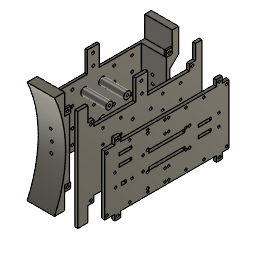
soccerbot (Autodesk Fusion 360 design; units mm, degrees)
part number: 2026-01-25-12-54-34-821
Autodesk Fusion 360 part; units mm, degrees
sketch "Sketch1" plane through (0, 0, 0) normal (1, 0, 0) x (0, 1, 0)
sketch "Base FL1" plane through (0, 0, 0) normal (1, 0, 0) x (0, 1, 0)
  line L0 (176.22, 50.0312) -> (1.6941, 50.0085) construction
  line L1 (90, 0) -> (90, 99.9394) construction
  line L2 (40, 22) -> (140, 22) construction
  line L3 (155, 34) -> (125, 34)
  line L4 (125, 34) -> (125, 10)
  line L5 (125, 10) -> (155, 10)
  line L6 (155, 10) -> (155, 34)
  line L7 (154.9958, 66.0568) -> (124.9958, 66.049)
  line L8 (124.9958, 66.049) -> (124.9896, 90.049)
  line L9 (124.9896, 90.049) -> (154.9896, 90.0568)
  line L10 (154.9896, 90.0568) -> (154.9958, 66.0568)
  line L11 (55, 34) -> (55, 10)
  line L12 (25, 34) -> (55, 34)
  line L13 (25, 10) -> (25, 34)
  line L14 (55, 10) -> (25, 10)
  line L15 (124.9896, 90.049) -> (154.9896, 90.0568)
  line L16 (124.9958, 66.049) -> (124.9896, 90.049)
  line L17 (154.9896, 90.0568) -> (154.9958, 66.0568)
  line L18 (154.9958, 66.0568) -> (124.9958, 66.049)
  line L19 (54.9896, 90.0308) -> (24.9896, 90.023)
  line L20 (54.9958, 66.0308) -> (54.9896, 90.0308)
  line L21 (24.9958, 66.023) -> (54.9958, 66.0308)
  line L22 (24.9896, 90.023) -> (24.9958, 66.023)
  line L23 (140, 10) -> (140, -25) construction
  line L24 (175, -25) -> (105, -25) construction
  line L25 (100, 0) -> (86, 0)
  line L26 (100, -35) -> (100, 0)
  line L27 (80, -35) -> (80, 0)
  line L28 (180, -35) -> (191, -35)
  line L29 (191, 135) -> (180, 135)
  line L30 (0, -36.9171) -> (-17, -36.8837)
  line L31 (5, -25) -> (75, -25) construction
  line L32 (191, 135) -> (191, 95)
  circle A0 centre (105, 22) radius 6
  circle A1 centre (75, 22) radius 6
  circle A2 centre (74.9927, 78.036) radius 6
  circle A3 centre (105.0073, 78.036) radius 6
  line L33 (180, 0) -> (0, 0)
  line L34 (176.2425, 80.55) -> (176.1975, 19.5123)
  line L35 (180, 0) -> (180, -35)
  line L36 (0, 0) -> (0, -36.9171)
  line L37 (180, 100) -> (0, 100)
  line L38 (180, 135) -> (180, 100)
  line L39 (176.1975, 19.5123) -> (191, 5)
  line L40 (191, 5) -> (191, -35)
  line L41 (191, 95) -> (176.2425, 80.55)
  line L42 (4.9805, 125.0178) -> (74.9805, 125.036) construction
  line L43 (174.9805, 125.062) -> (104.9805, 125.0438) construction
  line L44 (0, 100) -> (0, 135)
  line L45 (0, 135) -> (-17, 135)
  arc A4 (-17, -36.8837) -> (-17, 135) centre (-205.1779, 49.0581) ccw
  line L46 (8.1772, 100) -> (8.1772, 0)
  line L47 (170.3633, 100) -> (170.3633, 0)
  line L48 (100, 100) -> (100, 135)
  line L49 (80, 100) -> (80, 135)
  line L50 (100, 135) -> (80, 135)
  line L51 (80, -35) -> (100, -35)
  point P0 (90, 22)
  point P1 (40, 22)
  point P2 (39.9927, 78.0269)
  point P3 (39.9927, 78.0269)
  point P4 (176.1975, 19.5123)
  point P5 (191, 5)
  dimension "d2" = 180
  dimension "d31" = 30
  dimension "d32" = 30
  dimension "d33" = 24
  dimension "d36" = 35
  dimension "d46" = 17
  dimension "d47" = 11
  dimension "d51" = 12
  dimension "d53" = 11
  dimension "d59" = 35
  dimension "d63" = 35
  dimension "d64" = 17
  dimension "d65" = 35
  dimension "d66" = 35
  constraint midpoint L2 P0
  constraint coincident L1 P0
  constraint perpendicular L1 L2
  constraint horizontal L3
  constraint vertical L4
  constraint horizontal L5
  constraint vertical L6
  constraint symmetric L0 L3.start L7.start
  constraint symmetric L0 L3.end L7.end
  constraint symmetric L0 L4.end L8.end
  constraint symmetric L0 L5.end L9.end
  constraint symmetric L1 L2.end P1
  constraint symmetric L1 L3.start L12.start
  constraint symmetric L1 L3.end L11.start
  constraint symmetric L1 L4.end L11.end
  constraint symmetric L1 L5.end L13.start
  constraint symmetric L0 P1 P3
  constraint symmetric L0 L11.end L19.start
  constraint symmetric L0 L11.start L20.start
  constraint symmetric L0 L13.start L19.end
  constraint symmetric L0 L12.start L21.start
  constraint midpoint L5 L23.start
  constraint perpendicular L5 L23
  constraint midpoint L23.end L24
  constraint perpendicular L23 L24
  constraint horizontal L25
  constraint vertical L26
  constraint symmetric L1 L25.start L27.end
  constraint symmetric L1 L26.start L27.start
  constraint horizontal L28
  constraint horizontal L29
  constraint symmetric L1 L24.start L31.start
  constraint symmetric L1 L24.end L31.end
  constraint coincident L2 A0.centre
  constraint symmetric L1 A0 A1
  constraint symmetric L0 A1 A2
  constraint symmetric L1 A2 A3
  constraint coincident L33.end L36.start
  constraint vertical L36
  constraint horizontal L37
  constraint coincident P4 L34.end
  constraint coincident P5 L39.end
  constraint vertical L32
  constraint symmetric L0 L31.start L42.start
  constraint symmetric L0 L31.end L42.end
  constraint symmetric L0 L24.start L43.start
  constraint symmetric L0 L24.end L43.end
  constraint perpendicular L37 L44
  constraint perpendicular L44 L45
  constraint coincident L0.end A4
  constraint midpoint L0.start L34
  constraint coincident L37 L46.start
  constraint coincident L33 L46.end
  constraint perpendicular L33 L46
  constraint coincident L37 L47.start
  constraint coincident L33 L47.end
  constraint perpendicular L33 L47
  constraint coincident L37 L48.start
  constraint perpendicular L37 L48
  constraint coincident L37 L49.start
  constraint perpendicular L37 L49
  constraint perpendicular L26 L51
  measures "d2" distance of L33.end L33.start
  measures "d31" distance of L4.end L5.end
  measures "d32" distance of L3.start L3.end
  measures "d33" distance of L3.start L5.end
  measures "d36" distance of L25.start L26.start
  measures "d46" distance of L30.end L30.start
  measures "d47" distance of L28.start L28.end
  measures "d51" diameter of A0
  measures "d53" distance of L29.start L29.end
  measures "d59" distance of L33.start L28.start
  measures "d63" distance of L37.end L44.end
  measures "d64" distance of L44.end L45.end
  measures "d65" distance of L48.start L48.end
  measures "d66" distance of L49.start L49.end
extrude "Extrude4" add sketch "Base FL1" along normal blind 46 contours L28 L29 L32 L33 L34 L35 L37 L38 L39 L40 L41 L47 | L30 L33 L36 L37 L44 L45 A4 L46 | A0 | A1 | A2 | A3 makes body 1 at (30.6667, 69.0225, 77.4386) makes body 2 at (30.6667, 0.7595, 68.7236) makes body 3 at (30.6667, 80.9925, 21.7009) makes body 4 at (30.6667, 99.0371, 77.4386) makes body 5 at (30.6667, 170.3633, 66.6667) makes body 6 at (30.6667, 110.9925, 21.7009)
extrude "Extrude5" add sketch "Base FL1" along normal blind 4 contours L3 L4 L5 L6 | L7 L8 L9 L10 L15 L16 L17 L18 | L11 L12 L13 L14 | L19 L20 L21 L22 | L25 L26 L27 L33 L51 | L25 L33 L37 L46 L47 | L37 L48 L49 L50 bodies 1 2 3 4 5 6
hole "Hole3" at (0, 25, 10) at (0, 25, 34) at (0, 55, 34) at (0, 55, 10) at (0, 125, 34) at (0, 155, 34) at (0, 155, 10) at (0, 125, 10) at (0, 124.9896, 90.049) at (0, 154.9896, 90.0568) at (0, 154.9958, 66.0568) at (0, 124.9958, 66.049) at (0, 54.9958, 66.0308) at (0, 54.9896, 90.0308) at (0, 24.9896, 90.023) at (0, 24.9958, 66.023) direction (1, 0, 0) diameter 4.5 depth 4 tip angle 180 bodies 1
hole "Hole4" at (0, 74.9927, 78.036) at (0, 105.0073, 78.036) at (0, 105, 22) at (0, 75, 22) direction (1, 0, 0) diameter 3.783 depth 20 tip angle 180 bodies 1
thread "Thread1" "ISO Metric profile 4.5 M4.5x0.75 M4.5x0.75 6H" major diameter 4.6131 minor diameter 3.7831 pitch 0.75 angle 60 resizes the face on face at (6.6667, 106.5431, 76.9319) on face at (6.6667, 105.0943, 23.8891) on face at (6.6667, 76.5285, 76.9319) on face at (6.6667, 75.0943, 23.8891) on bodies 1
hole "Hole5" at (0, 74.9927, 78.036) at (0, 105.0073, 78.036) at (0, 105, 22) at (0, 75, 22) direction (1, 0, 0) diameter 3.783 depth 46 tip angle 180 bodies 1
thread "Thread2" "ISO Metric profile 4.5 M4.5x0.75 M4.5x0.75 6H" major diameter 4.6131 minor diameter 3.7831 pitch 0.75 angle 60 resizes the face on face at (28.6667, 75.1883, 23.8821) on face at (28.6667, 76.5816, 77.0098) on face at (28.6667, 105.1883, 23.8821) on face at (28.6667, 106.5962, 77.0098) on bodies 1
hole "Hole6" at (4, 89.3779, 126.1811) direction (-1, 0, 0) diameter 4.5 depth 4 tip angle 180 bodies 1
hole "Hole7" at (4, 90.0772, 107.2797) direction (-1, 0, 0) diameter 4.5 depth 4 tip angle 180 bodies 1
hole "Hole8" at (22.4648, 176.2297, 63.2035) direction (0, -1, 0.000737) diameter 4.5 depth 5.877 tip angle 180 bodies 1
hole "Hole9" at (23, 176.22, 50.0312) direction (0, -1, 0.000737) diameter 4.5 depth 5.877 tip angle 180 bodies 1
hole "Hole10" at (23.0599, 176.2099, 36.3846) direction (0, -1, 0.000737) diameter 4.5 depth 5.877 tip angle 180 bodies 1
hole "Hole11" at (15.3916, 74.9927, 76.1445) direction (0, 0, -1) diameter 4.5 depth 5.877 tip angle 180 bodies 1
hole "Hole12" at (11.1565, 105.0073, 76.1445) direction (0, 0, -1) diameter 4.5 depth 5.877 tip angle 180 bodies 1
hole "Hole13" at (23.1083, 8.1772, 51.0089) direction (0, -1, 0) diameter 4.5 depth 19 tip angle 180 bodies 1
hole "Hole14" at (22.5371, 8.1772, 33.9979) direction (0, -1, 0) diameter 4.5 depth 19 tip angle 180 bodies 1
hole "Hole15" at (22.1531, 8.1772, 69.5516) direction (0, -1, 0) diameter 4.5 depth 19 tip angle 180 bodies 1
hole "Hole16" at (4, 90.9402, 50.4012) direction (-1, 0, 0) diameter 4.5 depth 19 tip angle 180 bodies 1
hole "Hole17" at (4, 90.6117, -26.9418) direction (-1, 0, 0) diameter 4.5 depth 19 tip angle 180 bodies 1
hole "Hole18" at (4, 90.6117, -8.1238) direction (-1, 0, 0) diameter 4.5 depth 19 tip angle 180 bodies 1
sketch "Overhang 1" plane through (0, 0, 0) normal (0, 1, 0) x (-1, 0, 0)
  line L0 (0, 100) -> (0, 135)
  line L1 (0, 135) -> (-46, 135)
  line L2 (-46, 135) -> (-46, 100)
  line L3 (-46, 100) -> (0, 100)
  line L4 (-46, 110.0202) -> (-26, 110.0202)
  line L5 (-26, 100.0202) -> (-46, 100.0202)
  line L6 (-46, 100.0202) -> (-46, 110.0202)
  line L7 (-46, 110.0202) -> (-46, 109.0202)
  line L8 (-46, 100.0202) -> (-46, 101.0202)
  line L9 (-46, 100.0202) -> (-43, 100.0202)
  line L10 (-46, 100.0202) -> (-43, 100.0202)
  line L11 (-43, 100.0202) -> (-43, 110.0202)
  dimension "d124" = 20
  dimension "d125" = 10
  dimension "d126" = 1
  dimension "d127" = 1
  constraint horizontal L4
  constraint horizontal L5
  constraint vertical L6
  constraint coincident L2 L4.start
  constraint coincident L6 L7.end
  constraint coincident L6 L8.end
  constraint coincident L5 L9.end
  constraint coincident L4 L11.end
  constraint perpendicular L4 L11
  measures "d124" distance of L5.start L5.end
  measures "d125" distance of L4.start L5.end
  measures "d126" distance of L4.start L7.end
  measures "d127" distance of L5.end L8.end
extrude "Extrude6" add sketch "Overhang 1" along normal blind 10 separate body contours L2 L4 L5 L6 L7 L8 L9 L10 L11 makes body 7
sketch "Overhang 2" plane through (0, 0, 0) normal (0, 1, 0) x (-1, 0, 0)
  line L0 (0, -36.9171) -> (0, 0)
  line L1 (0, 0) -> (-46, 0)
  line L2 (-46, 0) -> (-46, -36.9171)
  line L3 (-46, -36.9171) -> (0, -36.9171)
  line L4 (-46, 0) -> (-43, 0)
  line L5 (-43, 0) -> (-43, -10)
  line L6 (-43, -10) -> (-46, -10)
  line L7 (-46, -10) -> (-46, 0)
  dimension "d130" = 10
  dimension "d131" = 3
  constraint horizontal L4
  constraint vertical L5
  constraint horizontal L6
  constraint vertical L7
  constraint coincident L1.end L2.start
  measures "d130" distance of L4.end L5.end
  measures "d131" distance of L5.end L6.end
extrude "Extrude7" add sketch "Overhang 2" along normal blind 10 separate body contours L1 L2 L4 L5 L6 L7 makes body 8
sketch "Overhang 3 - 4" plane through (0, 180, 0) normal (0, -1, 0) x (1, 0, 0)
  line L0 (0, 135) -> (0, 100)
  line L1 (0, 100) -> (46, 100)
  line L2 (46, 100) -> (46, 135)
  line L3 (46, 135) -> (0, 135)
  line L4 (46, 110.1305) -> (46, 100.1305)
  line L5 (46, -10) -> (46, 0)
  line L6 (46, 0) -> (43, 0)
  line L7 (43, 0) -> (43, -10)
  line L8 (43, -10) -> (46, -10)
  line L9 (46, -10) -> (46, 0)
  line L10 (46, 100) -> (43, 100)
  line L11 (43, 100) -> (43, 110)
  line L12 (43, 110) -> (46, 110)
  line L13 (46, 110) -> (46, 100)
  point P0 (46, 0)
  dimension "d144" = 10
  dimension "d145" = 3
  constraint vertical L4
  constraint coincident L2 L4.end
  constraint vertical L5
  constraint horizontal L6
  constraint vertical L7
  constraint horizontal L8
  constraint vertical L9
  constraint coincident P0 L5.end
  constraint horizontal L10
  constraint vertical L11
  constraint horizontal L12
  constraint vertical L13
  constraint coincident L1.end L2.start
  measures "d144" distance of L1.end L12.end
  measures "d145" distance of L1.end L10.end
extrude "Extrude8" add sketch "Overhang 3 - 4" along normal blind 10 separate body contours L5 L6 L7 L8 L9 makes body 9
extrude "Extrude10" add sketch "Overhang 3 - 4" along normal blind 10 separate body contours L1 L2 L4 L10 L11 L12 L13 makes body 10
hole "Hole19" at (46, 174.9154, 104.8549) direction (-1, 0, 0) diameter 4.5 end through all bodies 10
hole "Hole20" at (46, 175.0929, -5) direction (-1, 0, 0) diameter 4.5 depth 3 tip angle 180 bodies 9
hole "Hole21" at (46, 5, -4.7674) direction (-1, 0, 0) diameter 4.5 depth 3 tip angle 180 bodies 8
hole "Hole22" at (46, 5, 105.2643) direction (-1, 0, 0) diameter 4.5 depth 3 tip angle 180 bodies 7
sketch "Base FL2" plane through (0, 0, 0) normal (1, 0, 0) x (0, 1, 0)
  line L0 (55, 34) -> (55, 10)
  line L1 (191, 50) -> (-17, 50) construction
  line L2 (55, 10) -> (25, 10)
  line L3 (25, 10) -> (25, 34)
  line L4 (124.9896, 90.049) -> (154.9896, 90.0568)
  line L5 (80, 100) -> (80, 135)
  line L6 (100, -35) -> (100, 0)
  line L7 (154.9896, 90.0568) -> (154.9958, 66.0568)
  line L8 (25, 34) -> (55, 34)
  line L9 (54.9896, 90.0308) -> (24.9896, 90.023)
  line L10 (125, 10) -> (155, 10)
  line L11 (154.9958, 66.0568) -> (124.9958, 66.049)
  line L12 (154.9958, 66.0568) -> (124.9958, 66.049)
  line L13 (54.9958, 66.0308) -> (54.9896, 90.0308)
  line L14 (154.9896, 90.0568) -> (154.9958, 66.0568)
  line L15 (100, 135) -> (80, 135)
  line L16 (24.9896, 90.023) -> (24.9958, 66.023)
  line L17 (155, 10) -> (155, 34)
  line L18 (180, 0) -> (180, -35)
  line L19 (100, 100) -> (100, 135)
  line L20 (125, 34) -> (125, 10)
  line L21 (180, -35) -> (191, -35)
  line L22 (124.9896, 90.049) -> (154.9896, 90.0568)
  line L23 (124.9958, 66.049) -> (124.9896, 90.049)
  line L24 (180, 135) -> (180, 100)
  line L25 (124.9958, 66.049) -> (124.9896, 90.049)
  line L26 (80, -35) -> (100, -35)
  line L27 (80, -35) -> (80, 0)
  line L28 (24.9958, 66.023) -> (54.9958, 66.0308)
  line L29 (0, 135) -> (0, 100)
  line L30 (170, 0) -> (170, -10)
  line L31 (170, -10) -> (180, -10)
  line L32 (191, -35) -> (191, 135)
  line L33 (191, 135) -> (180, 135)
  line L34 (180, 135) -> (180, 110)
  line L35 (170, 100) -> (170, 110)
  line L36 (170, 110) -> (180, 110)
  line L37 (0, 110) -> (10, 110)
  line L38 (10, 110) -> (10, 100)
  line L39 (125, 34) -> (125, 10)
  line L40 (155, 10) -> (155, 34)
  line L41 (0, 135) -> (-17, 135)
  line L42 (125, 34) -> (155, 34)
  line L43 (180, 100) -> (100, 100)
  line L44 (0, 100) -> (80, 100)
  line L45 (0, 0) -> (80, 0)
  line L46 (0, 0.2133) -> (0, -34.7867)
  line L47 (0, -34.7867) -> (-17, -34.7867)
  line L48 (-17, 135) -> (-17, -34.7867)
  line L49 (180, 0) -> (100, 0)
  line L50 (0, -10) -> (10, -10)
  line L51 (10, -10) -> (10, 0)
  line L52 (24.9927, 59.9133) -> (55, 59.9133)
  line L53 (55, 59.9133) -> (55, 40)
  line L54 (55, 40) -> (24.9927, 40)
  line L55 (24.9927, 40) -> (24.9927, 59.9133)
  line L56 (90, 135) -> (90, -35) construction
  line L57 (155.0073, 59.9133) -> (125, 59.9133)
  line L58 (125, 59.9133) -> (125, 40)
  line L59 (125, 40) -> (155.0073, 40)
  line L60 (155.0073, 40) -> (155.0073, 59.9133)
  circle A0 centre (105.0073, 78.036) radius 6
  circle A1 centre (105.0073, 21.964) radius 6
  circle A2 centre (74.9927, 21.964) radius 6
  line L61 (180, 0) -> (180, -35)
  line L62 (155, 10) -> (155, 34)
  line L63 (155.0073, 40) -> (155.0073, 59.9133)
  line L64 (-17, 135) -> (-17, -34.7867)
  line L65 (80, -35) -> (100, -35)
  line L66 (54.9896, 90.0308) -> (24.9896, 90.023)
  line L67 (55, 10) -> (25, 10)
  line L68 (155, 10) -> (155, 34)
  line L69 (125, 40) -> (155.0073, 40)
  line L70 (170, 0) -> (170, -10)
  line L71 (24.9927, 59.9133) -> (55, 59.9133)
  line L72 (155.0073, 59.9133) -> (125, 59.9133)
  line L73 (154.9958, 66.0568) -> (124.9958, 66.049)
  line L74 (124.9896, 90.049) -> (154.9896, 90.0568)
  line L75 (124.9896, 90.049) -> (154.9896, 90.0568)
  line L76 (124.9958, 66.049) -> (124.9896, 90.049)
  line L77 (0, 135) -> (0, 100)
  line L78 (25, 34) -> (55, 34)
  line L79 (0, 110) -> (10, 110)
  line L80 (154.9896, 90.0568) -> (154.9958, 66.0568)
  line L81 (180, 135) -> (180, 100)
  line L82 (125, 34) -> (125, 10)
  line L83 (170, -10) -> (180, -10)
  line L84 (124.9958, 66.049) -> (124.9896, 90.049)
  line L85 (0, 0) -> (80, 0)
  line L86 (191, 135) -> (180, 135)
  line L87 (10, 110) -> (10, 100)
  line L88 (80, -35) -> (80, 0)
  line L89 (0, 100) -> (80, 100)
  line L90 (0, 135) -> (-17, 135)
  line L91 (100, -35) -> (100, 0)
  line L92 (55, 40) -> (24.9927, 40)
  line L93 (125, 10) -> (155, 10)
  line L94 (170, 100) -> (170, 110)
  line L95 (154.9958, 66.0568) -> (124.9958, 66.049)
  line L96 (125, 34) -> (155, 34)
  line L97 (125, 34) -> (125, 10)
  line L98 (170, 110) -> (180, 110)
  line L99 (24.9958, 66.023) -> (54.9958, 66.0308)
  line L100 (55, 34) -> (55, 10)
  line L101 (180, -35) -> (191, -35)
  line L102 (180, 135) -> (180, 110)
  line L103 (80, 100) -> (80, 135)
  line L104 (100, 100) -> (100, 135)
  circle A3 centre (74.9927, 78.036) radius 6
  line L105 (100, 135) -> (80, 135)
  line L106 (24.9896, 90.023) -> (24.9958, 66.023)
  line L107 (54.9958, 66.0308) -> (54.9896, 90.0308)
  line L108 (191, 50) -> (-17, 50) construction
  line L109 (25, 10) -> (25, 34)
  line L110 (10, -10) -> (10, 0)
  line L111 (0, 0.2133) -> (0, -34.7867)
  line L112 (180, 0) -> (100, 0)
  line L113 (0, -10) -> (10, -10)
  line L114 (0, -34.7867) -> (-17, -34.7867)
  line L115 (125, 59.9133) -> (125, 40)
  line L116 (90, 135) -> (90, -35) construction
  line L117 (191, -35) -> (191, 135)
  line L118 (180, 100) -> (100, 100)
  line L119 (24.9927, 40) -> (24.9927, 59.9133)
  line L120 (55, 59.9133) -> (55, 40)
  circle A4 centre (25, 34) radius 2
  circle A5 centre (25, 10) radius 2
  circle A6 centre (55, 34) radius 2
  circle A7 centre (55, 10) radius 2
  circle A8 centre (24.9896, 90.023) radius 2
  circle A9 centre (54.9896, 90.0308) radius 2
  circle A10 centre (54.9958, 66.0308) radius 2
  circle A11 centre (24.9958, 66.023) radius 2
  circle A12 centre (74.9927, 21.964) radius 6
  circle A13 centre (105.0073, 21.964) radius 6
  circle A14 centre (105.0073, 78.036) radius 6
  circle A15 centre (74.9927, 78.036) radius 6
  circle A16 centre (124.9958, 66.049) radius 2
  circle A17 centre (154.9958, 66.0568) radius 2
  circle A18 centre (154.9896, 90.0568) radius 2
  circle A19 centre (124.9896, 90.049) radius 2
  circle A20 centre (155, 34) radius 2
  circle A21 centre (155, 10) radius 2
  circle A22 centre (125, 10) radius 2
  circle A23 centre (125, 34) radius 2
  dimension "d237" = 4
  dimension "d238" = 4
  dimension "d239" = 4
  dimension "d240" = 4
  dimension "d241" = 4
  dimension "d242" = 4
  dimension "d243" = 4
  dimension "d244" = 4
  dimension "d245" = 12
  dimension "d246" = 12
  dimension "d247" = 12
  dimension "d248" = 4
  dimension "d249" = 4
  dimension "d250" = 4
  dimension "d251" = 4
  dimension "d252" = 4
  dimension "d253" = 4
  dimension "d254" = 4
  dimension "d255" = 4
  constraint coincident L18 L31.end
  constraint coincident L24 L34.end
  constraint coincident L29 L37.start
  constraint perpendicular L29 L37
  constraint perpendicular L17 L42
  constraint midpoint L1.start L32
  constraint coincident L45.start L85.start
  constraint perpendicular L27 L45
  constraint perpendicular L45 L46
  constraint perpendicular L46 L47
  constraint perpendicular L6 L49
  constraint coincident L46 L50.start
  constraint perpendicular L46 L50
  constraint coincident L45 L51.end
  constraint perpendicular L45 L51
  constraint horizontal L52
  constraint vertical L53
  constraint horizontal L54
  constraint vertical L55
  constraint midpoint L15 L56.start
  constraint midpoint L26 L56.end
  constraint symmetric L52.start L56 L57.start
  constraint symmetric L52.end L56 L57.end
  constraint symmetric L53.end L56 L58.end
  constraint symmetric L54.end L56 L59.end
  constraint symmetric L1 A0 A1
  constraint symmetric L56 A1 A2
  constraint coincident L31.end L61
  constraint coincident L34.end L81
  constraint coincident L37.start L77
  constraint perpendicular L77 L79
  constraint perpendicular L68 L96
  constraint midpoint L1.start L117
  constraint perpendicular L85 L88
  constraint perpendicular L85 L111
  constraint perpendicular L111 L114
  constraint perpendicular L91 L112
  constraint coincident L50.start L111
  constraint perpendicular L111 L113
  constraint coincident L51.end L85
  constraint perpendicular L85 L110
  constraint horizontal L71
  constraint vertical L120
  constraint horizontal L92
  constraint vertical L119
  constraint midpoint L56.start L105
  constraint midpoint L56.end L65
  constraint symmetric L57.start L52.start L116
  constraint symmetric L57.end L52.end L116
  constraint symmetric L58.end L53.end L116
  constraint symmetric L54.end L59.end L116
  constraint coincident L3.end L8.start
  constraint coincident L2.end L3.start
  constraint coincident L0.start L8.end
  constraint coincident L0.end L2.start
  constraint coincident L9.end L16.start
  constraint coincident L9.start L13.end
  constraint coincident L13.start L28.end
  constraint coincident L16.end L28.start
  constraint concentric A2 A12
  constraint concentric A1 A13
  constraint concentric A0 A14
  constraint concentric A3 A15
  constraint coincident L11.end L12.end
  constraint coincident L7.end L11.start
  constraint coincident L4.end L7.start
  constraint coincident L4.start L22.start
  constraint coincident L17.end L40.end
  constraint coincident L10.end L17.start
  constraint coincident L10.start L20.end
  constraint coincident L20.start L39.start
  measures "d237" diameter of A7
  measures "d238" diameter of A6
  measures "d239" diameter of A4
  measures "d240" diameter of A5
  measures "d241" diameter of A11
  measures "d242" diameter of A8
  measures "d243" diameter of A9
  measures "d244" diameter of A10
  measures "d245" diameter of A14
  measures "d246" diameter of A13
  measures "d247" diameter of A12
  measures "d248" diameter of A22
  measures "d249" diameter of A21
  measures "d250" diameter of A20
  measures "d251" diameter of A23
  measures "d252" diameter of A16
  measures "d253" diameter of A17
  measures "d254" diameter of A18
  measures "d255" diameter of A19
sketch "Sketch8" plane through (55, 0, 0) normal (1, 0, 0) x (0, 1, 0)
extrude "Extrude12" add sketch "Base FL2" along normal blind 5 separate body contours L0 L2 L3 L8 L67 L78 L100 L109 A4 A5 A6 A7 | L4 L7 L11 L12 L14 L22 L23 L25 L73 L74 L75 L76 L80 L84 L95 A16 A17 A18 A19 | L5 L6 L15 L18 L19 L21 L24 L26 L27 L29 L32 L33 L34 L41 L43 L44 L45 L46 L47 L48 L49 L61 L64 L65 L77 L81 L85 L86 L88 L89 L90 L91 L101 L102 L103 L104 L105 L111 L112 L114 L117 L118 | L29 L37 L38 L44 L77 L79 L87 L89 | L24 L35 L36 L43 L81 L94 L98 L118 | L45 L46 L50 L51 L85 L110 L111 L113 | L18 L30 L31 L49 L61 L70 L83 L112 | L9 L13 L16 L28 L66 L99 L106 L107 A8 A9 A10 A11 | L10 L17 L20 L39 L40 L42 L62 L68 L82 L93 L96 L97 A20 A21 A22 A23 | A0 A14 | A1 A13 | A2 A12 | A3 A15 makes body 11
hole "Hole35" at (0, 74.9927, 78.036) direction (1, 0, 0) diameter 4.5 depth 5 tip angle 180 bodies 11
hole "Hole36" at (0, 105.0073, 78.036) direction (1, 0, 0) diameter 4.5 depth 5 tip angle 180 bodies 11
hole "Hole37" at (0, 105.0073, 21.964) direction (1, 0, 0) diameter 4.5 depth 5 tip angle 180 bodies 11
hole "Hole38" at (0, 74.9927, 21.964) direction (1, 0, 0) diameter 4.5 depth 5 tip angle 180 bodies 11
move_body "Move2" bodies 11 to x (1, 0, 0) y (0, 1, 0) z (0, 0, 1) at (50, 0, 0)
hole "Hole39" at (50, 174.9118, 104.9201) direction (1, 0, 0) diameter 4.5 depth 5 tip angle 180 bodies 11
hole "Hole40" at (50, 175.1424, -5.038) direction (1, 0, 0) diameter 4.5 depth 5 tip angle 180 bodies 11
hole "Hole41" at (50, 90.3269, -8.1207) direction (1, 0, 0) diameter 4.5 depth 5 tip angle 180 bodies 11
hole "Hole42" at (50, 90.6224, -26.9185) direction (1, 0, 0) diameter 4.5 depth 5 tip angle 180 bodies 11
hole "Hole43" at (50, 90.9577, 50.4083) direction (1, 0, 0) diameter 4.5 depth 5 tip angle 180 bodies 11
hole "Hole44" at (50, 89.3921, 126.1895) direction (1, 0, 0) diameter 4.5 depth 5 tip angle 180 bodies 11
hole "Hole45" at (50, 90.0893, 107.3095) direction (1, 0, 0) diameter 4.5 depth 5 tip angle 180 bodies 11
hole "Hole46" at (50, 5.0185, -4.7346) direction (1, 0, 0) diameter 4.5 depth 5 tip angle 180 bodies 11
hole "Hole47" at (50, 5.0143, 105.2605) direction (1, 0, 0) diameter 4.5 depth 5 tip angle 180 bodies 11
sketch "Sketch9" plane through (55, 0, 0) normal (1, 0, 0) x (0, 1, 0)
  line L0 (-17.0199, 0) -> (190.9801, 0)
  line L1 (190.9801, 0) -> (190.9801, 100)
  line L2 (190.9801, 100) -> (-17.0199, 100)
  line L3 (-17.0199, 100) -> (-17.0199, 0)
  line L4 (0, 100) -> (10, 100)
  line L5 (10, 100) -> (10, 110)
  line L6 (10, 110) -> (0, 110)
  line L7 (0, 110) -> (0, 100)
  line L8 (0, 0) -> (10, 0)
  line L9 (10, 0) -> (10, -10)
  line L10 (10, -10) -> (0, -10)
  line L11 (0, -10) -> (0, 0)
  line L12 (180, 0) -> (170, 0)
  line L13 (170, 0) -> (170, -10)
  line L14 (170, -10) -> (180, -10)
  line L15 (180, -10) -> (180, 0)
  line L16 (180, 100) -> (170, 100)
  line L17 (170, 100) -> (170, 110)
  line L18 (170, 110) -> (180, 110)
  line L19 (180, 110) -> (180, 100)
  circle A0 centre (90, 25) radius 2
  circle A1 centre (90, 75) radius 2
  circle A2 centre (0.0264, 60.0061) radius 2
  circle A3 centre (-13, 95) radius 2
  circle A4 centre (25, 95) radius 2
  circle A5 centre (55, 95) radius 2
  circle A6 centre (84, 95) radius 2
  line L20 (-17.0199, 50) -> (190.9801, 50) construction
  line L21 (86.9801, 100) -> (86.9801, 0) construction
  circle A7 centre (84, 75) radius 2
  circle A8 centre (84, 25) radius 2
  circle A9 centre (89.9602, 95) radius 2
  circle A10 centre (118.9602, 95) radius 2
  circle A11 centre (118.9602, 66) radius 2
  circle A12 centre (148.9602, 95) radius 2
  circle A13 centre (173.9337, 60.0061) radius 2
  circle A14 centre (186.9602, 95) radius 2
  circle A15 centre (173.9337, 39.9939) radius 2
  circle A16 centre (186.9602, 5) radius 2
  circle A17 centre (148.9602, 5) radius 2
  circle A18 centre (118.9602, 5) radius 2
  circle A19 centre (118.9602, 34) radius 2
  circle A20 centre (84, 5) radius 2
  circle A21 centre (89.9602, 5) radius 2
  circle A22 centre (55, 5) radius 2
  circle A23 centre (25, 5) radius 2
  circle A24 centre (-13, 5) radius 2
  line L22 (56.9801, 35.0016) -> (116.9801, 35.0016)
  line L23 (116.9801, 35.0016) -> (116.9801, 40.0016)
  line L24 (116.9801, 40.0016) -> (57, 40.0016)
  line L25 (57, 40.0016) -> (56.9801, 35.0016)
  line L26 (56.99, 37.5016) -> (116.9801, 37.5016) construction
  circle A25 centre (47.4401, 61.75) radius 2
  circle A26 centre (47.4401, 38.25) radius 2
  line L27 (56.9801, 62.625) -> (116.9801, 62.625) construction
  line L28 (56.9801, 65.125) -> (56.9801, 60.125)
  line L29 (56.9801, 60.125) -> (116.9801, 60.125)
  line L30 (56.9801, 65.125) -> (116.9801, 65.125)
  line L31 (116.9801, 65.125) -> (116.9801, 60.125)
  line L32 (7.2113, 85.4863) -> (28.2113, 85.4863)
  line L33 (7.2113, 64.4863) -> (28.2113, 64.4863)
  line L34 (28.2113, 85.4863) -> (7.2113, 85.4863)
  line L35 (7.2113, 80.9863) -> (28.2113, 80.9863)
  line L36 (28.2113, 68.9863) -> (7.2113, 68.9863)
  line L37 (28.2113, 80.9863) -> (28.2113, 85.4863)
  line L38 (28.2113, 68.9863) -> (28.2113, 64.4863)
  line L39 (7.2113, 85.4863) -> (7.2113, 80.9863)
  line L40 (7.2113, 68.9863) -> (7.2113, 64.4863)
  line L41 (139.9602, 60.5) -> (160.9602, 60.5)
  line L42 (139.9602, 56) -> (139.9602, 60.5)
  line L43 (160.9602, 56) -> (139.9602, 56)
  line L44 (160.9602, 60.5) -> (160.9602, 56)
  line L45 (139.9602, 44) -> (160.9602, 44)
  line L46 (160.9602, 44) -> (160.9602, 39.5)
  line L47 (160.9602, 39.5) -> (139.9602, 39.5)
  line L48 (139.9602, 44) -> (139.9602, 39.5)
  line L49 (11, 41) -> (19, 41)
  line L50 (19, 41) -> (19, 36)
  line L51 (19, 36) -> (11, 36)
  line L52 (11, 36) -> (11, 41)
  line L53 (19, 38.5) -> (11, 38.5) construction
  circle A27 centre (28.75, 38) radius 2
  line L54 (15, 41) -> (15, 36) construction
  circle A28 centre (1.25, 38) radius 2
  point P0 (89.9602, 95)
  point P1 (118.9602, 95)
  point P2 (118.9602, 66)
  point P3 (148.9602, 95)
  point P4 (173.9337, 60.0061)
  point P5 (186.9602, 95)
  point P6 (-13, 5)
  point P7 (25, 5)
  point P8 (10, 34)
  point P9 (55, 34)
  point P10 (55, 5)
  point P11 (84, 5)
  point P12 (89.9602, 5)
  point P13 (90, 25)
  point P14 (118.9602, 34)
  point P15 (118.9602, 5)
  point P16 (148.9602, 5)
  point P17 (173.9337, 39.9939)
  point P18 (84, 5)
  point P19 (186.9602, 5)
  point P20 (86.9801, 35.0016)
  point P21 (86.9801, 50)
  point P22 (47.4401, 50)
  point P23 (-2, 50)
  point P24 (3, 50)
  point P25 (1.25, 38)
  dimension "d315" = 4
  dimension "d317" = 4
  dimension "d318" = 4
  dimension "d319" = 4
  dimension "d320" = 4
  dimension "d321" = 4
  dimension "d326" = 4
  dimension "d329" = 4
  dimension "d330" = 4
  dimension "d331" = 4
  dimension "d332" = 4
  dimension "d333" = 4
  dimension "d334" = 4
  dimension "d335" = 4
  dimension "d336" = 4
  dimension "d337" = 4
  dimension "d338" = 4
  dimension "d339" = 4
  dimension "d340" = 4
  dimension "d341" = 4
  dimension "d342" = 4
  dimension "d343" = 4
  dimension "d344" = 4
  dimension "d345" = 4
  dimension "d347" = 60
  dimension "d348" = 5
  dimension "d353" = 4
  dimension "d354" = 4
  dimension "d368" = 4
  dimension "d369" = 4
  constraint horizontal L0
  constraint vertical L1
  constraint horizontal L2
  constraint vertical L3
  constraint horizontal L4
  constraint vertical L5
  constraint horizontal L6
  constraint vertical L7
  constraint coincident L2 L4.start
  constraint horizontal L8
  constraint vertical L9
  constraint horizontal L10
  constraint vertical L11
  constraint coincident L8.start L11.end
  constraint horizontal L12
  constraint vertical L13
  constraint horizontal L14
  constraint vertical L15
  constraint coincident L0 L12.start
  constraint horizontal L16
  constraint vertical L17
  constraint horizontal L18
  constraint vertical L19
  constraint coincident L2 L16.start
  constraint midpoint L3 L20.start
  constraint midpoint L1 L20.end
  constraint midpoint L2 L21.start
  constraint midpoint L0 L21.end
  constraint symmetric A2.centre L21 P4
  constraint symmetric A3.centre L21 P5
  constraint symmetric A4.centre L21 P3
  constraint symmetric A5.centre L21 P1
  constraint symmetric A6.centre L21 P0
  constraint symmetric A1.centre L20 P13
  constraint symmetric A3.centre L20 P6
  constraint symmetric A4.centre L20 P7
  constraint symmetric A5.centre L20 P10
  constraint symmetric A6.centre L20 P18
  constraint symmetric L20 P0 P12
  constraint symmetric L20 P1 P15
  constraint symmetric L20 P2 P14
  constraint symmetric L20 P3 P16
  constraint symmetric L20 P4 P17
  constraint symmetric L20 A7 A8
  constraint symmetric L20 P5 P19
  constraint coincident P0 A9.centre
  constraint coincident P1 A10.centre
  constraint coincident P2 A11.centre
  constraint coincident P3 A12.centre
  constraint coincident P4 A13.centre
  constraint coincident P5 A14.centre
  constraint coincident P17 A15.centre
  constraint coincident P19 A16.centre
  constraint coincident P16 A17.centre
  constraint coincident P15 A18.centre
  constraint coincident P14 A19.centre
  constraint coincident P18 P11
  constraint coincident P12 A21.centre
  constraint coincident P10 A22.centre
  constraint coincident P7 A23.centre
  constraint coincident P6 A24.centre
  constraint midpoint L22 P20
  constraint coincident L21 P20
  constraint perpendicular L21 L22
  constraint perpendicular L22 L23
  constraint perpendicular L21 L24
  constraint midpoint L25 L26.start
  constraint midpoint L23 L26.end
  constraint coincident L20 P21
  constraint coincident L20 P22
  constraint midpoint L27.start L28
  constraint perpendicular L27 L28
  constraint perpendicular L21 L30
  constraint perpendicular L29 L31
  constraint coincident L20 P23
  constraint horizontal L33
  constraint horizontal L34
  constraint coincident L20 P24
  constraint horizontal L35
  constraint horizontal L36
  constraint perpendicular L35 L39
  constraint perpendicular L33 L40
  constraint horizontal L49
  constraint vertical L50
  constraint horizontal L51
  constraint vertical L52
  constraint midpoint L50 L53.start
  constraint midpoint L52 L53.end
  constraint midpoint L49 L54.start
  constraint midpoint L51 L54.end
  constraint symmetric A27.centre L54 P25
  constraint coincident P25 A28.centre
  measures "d315" diameter of A1
  measures "d317" diameter of A2
  measures "d318" diameter of A3
  measures "d319" diameter of A4
  measures "d320" diameter of A5
  measures "d321" diameter of A6
  measures "d326" diameter of A0
  measures "d329" diameter of A7
  measures "d330" diameter of A9
  measures "d331" diameter of A10
  measures "d332" diameter of A11
  measures "d333" diameter of A12
  measures "d334" diameter of A13
  measures "d335" diameter of A14
  measures "d336" diameter of A15
  measures "d337" diameter of A16
  measures "d338" diameter of A17
  measures "d339" diameter of A18
  measures "d340" diameter of A19
  measures "d341" diameter of A20
  measures "d342" diameter of A21
  measures "d343" diameter of A22
  measures "d344" diameter of A23
  measures "d345" diameter of A24
  measures "d347" distance of L22.start L22.end
  measures "d348" distance of L22.end L23.end
  measures "d353" diameter of A25
  measures "d354" diameter of A26
  measures "d368" diameter of A27
  measures "d369" diameter of A28
extrude "Extrude13" add sketch "Sketch9" along normal blind 5 separate body makes body 12
move_body "Move3" bodies 12 to x (1, 0, 0) y (0, 1, 0) z (0, 0, 1) at (70, 0, 0)
move_body "Move4" bodies 11 to x (1, 0, 0) y (0, 1, 0) z (0, 0, 1) at (10, 0, 0)
move_body "Move5" bodies 11 to x (1, 0, 0) y (0, 1, 0) z (0, 0, 1) at (30, 0, 0)
move_body "Move6" bodies 11 to x (1, 0, 0) y (0, 1, 0) z (0, 0, 1) at (-10, 0, 0)
hole "Hole48" at (125, 124.9842, 66.0428) direction (1, 0, 0) diameter 4.5 depth 5 tip angle 180 bodies 12
hole "Hole49" at (125, 125.0024, 34.0368) direction (1, 0, 0) diameter 4.5 depth 5 tip angle 180 bodies 12
hole "Hole50" at (125, 5.0525, -4.7081) direction (1, 0, 0) diameter 4.5 depth 5 tip angle 180 bodies 12
hole "Hole51" at (125, 5.0497, 105.3153) direction (1, 0, 0) diameter 4.5 depth 5 tip angle 180 bodies 12
hole "Hole52" at (125, 55.0248, 90.0621) direction (1, 0, 0) diameter 4.5 depth 5 tip angle 180 bodies 12
hole "Hole53" at (125, 54.9929, 10.027) direction (1, 0, 0) diameter 4.5 depth 5 tip angle 180 bodies 12
hole "Hole54" at (125, 175.1674, -4.9317) direction (1, 0, 0) diameter 4.5 depth 5 tip angle 180 bodies 12
hole "Hole55" at (125, 174.896, 104.9118) direction (1, 0, 0) diameter 4.5 depth 5 tip angle 180 bodies 12
hole "Hole56" at (125, 54.9396, 66.1043) direction (1, 0, 0) diameter 4.5 depth 5 tip angle 180 bodies 12
hole "Hole57" at (125, 54.9999, 34.0554) direction (1, 0, 0) diameter 4.5 depth 5 tip angle 180 bodies 12
ref_plane "WorkPlane1" through (-46, 0, 0) normal (1, 0, 0) x (0, 1, 0)
ref_plane "WorkPlane2" through (0, 0, 0) normal (1, 0, 0) x (0, 1, 0)
named bodies: "FL1", "Overhang 1", "Overhang 2", "Overhang 4", "Overhang 5", "FL2", "FL3"
